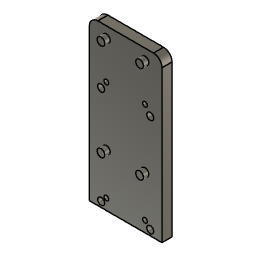
scope-strut-flange v6 (Autodesk Fusion 360 design; units mm, degrees)
Autodesk Fusion 360 part; units mm, degrees
note: some values were not read from the file. Set by a fixed rule: which sketch regions a step uses.
sketch "Sketch1" plane through (0, 0, 0) normal (0, 1, 0) x (1, 0, 0)
  line L0 (47, -103.5) -> (-36, -103.5)
  line L1 (-47, -103.5) -> (-47, 103.5)
  line L2 (-47, 103.5) -> (47, 103.5)
  line L3 (47, 103.5) -> (47, -103.5)
  line L4 (47, -103.5) -> (-47, 103.5) construction
  line L5 (-47, -103.5) -> (47, 103.5) construction
  line L6 (-47, -103.5) -> (36, -103.5)
  line L7 (47, -92.5) -> (47, 96.5)
  line L8 (47, 96.5) -> (-47, 96.5)
  line L9 (-47, 96.5) -> (-47, -92.5)
  line L10 (0, 96.5) -> (-31.75, 96.5)
  line L11 (-31.75, 96.5) -> (31.75, 96.5)
  line L12 (31.75, 96.5) -> (31.75, -30.5)
  line L13 (31.75, -30.5) -> (-31.75, -30.5)
  line L14 (-31.75, -30.5) -> (-31.75, 96.5)
  circle A0 centre (31.75, -30.5) radius 2.05
  circle A1 centre (-31.75, -30.5) radius 2.05
  circle A2 centre (31.75, 96.5) radius 2.05
  circle A3 centre (-31.75, 96.5) radius 2.05
  arc A4 (-47, -92.5) -> (-36, -103.5) centre (-36, -92.5) ccw
  arc A5 (36, -103.5) -> (47, -92.5) centre (36, -92.5) ccw
  point P0 (47, -103.5)
  dimension "d1" = 94
  dimension "d2" = 207
  dimension "d3" = 94
  dimension "d4" = 200
  dimension "d5" = 31.75
  dimension "d6" = 63.5
  dimension "d7" = 127
  dimension "d8" = 4.1
  dimension "d9" = 4.1
  dimension "d10" = 4.1
  dimension "d11" = 4.1
  dimension "d12" = 11
  constraint horizontal L0
  constraint perpendicular L0 L1
  constraint parallel L0 L2
  constraint parallel L1 L3
  constraint coincident L4 origin
  constraint coincident L5 origin
  constraint horizontal L6
  constraint vertical L7
  constraint horizontal L8
  constraint vertical L9
  constraint midpoint L8 L10.start
  constraint perpendicular L1 L10
  constraint horizontal L11
  constraint vertical L12
  constraint horizontal L13
  constraint vertical L14
  constraint coincident L12.end L13.start
  constraint coincident L13.end L14.start
  constraint coincident L11.end L12.start
  constraint coincident L10.end L11.start
  constraint coincident L1.start L0
  constraint coincident L1.start L9
  constraint tangent L0 A4
  constraint tangent L9 A4
  constraint coincident P0 L6
  constraint coincident P0 L7
  constraint tangent L6 A5
  constraint tangent L7 A5
  constraint equal A4 A5
  measures "d1" distance of L1.end L2.end
  measures "d2" distance of L1.start L1.end
  measures "d3" distance of L1.start P0
  measures "d4" distance of L1.start L8.end
  measures "d5" distance of L10.start L10.end
  measures "d6" distance of L10.end L11.end
  measures "d7" distance of L10.end L13.end
  measures "d8" diameter of A0
  measures "d9" diameter of A1
  measures "d10" diameter of A2
  measures "d11" diameter of A3
  measures "d12" radius of A4
extrude "Extrude1" add sketch "Sketch1" along normal blind 10 contours L0 L1 L3 L6 L7 L8 L9 L12 L13 L14 A0 A1 A2 A3 A4 A5 | L1 L2 L3 L8 L10 L11 A2 A3 | L8 L10 L11 L12 L13 L14 A0 A1 A2 A3
sketch "Sketch2" plane through (0, 0, 0) normal (0, -1, 0) x (1, 0, 0)
  circle A0 centre (31.75, -96.5) radius 2.05
  circle A1 centre (-31.75, -96.5) radius 2.05
  circle A2 centre (31.75, 30.5) radius 2.05
  circle A3 centre (-31.75, 30.5) radius 2.05
  line L0 (-47, 92.5) -> (-47, -103.5)
  line L1 (-47, -103.5) -> (47, -103.5)
  line L2 (47, -103.5) -> (47, 92.5)
  arc A4 (47, 92.5) -> (36, 103.5) centre (36, 92.5) ccw
  line L3 (36, 103.5) -> (-36, 103.5)
  arc A5 (-36, 103.5) -> (-47, 92.5) centre (-36, 92.5) ccw
  circle A6 centre (-31.75, 30.5) radius 4.5
  circle A7 centre (31.75, 30.5) radius 4.5
  circle A8 centre (-31.75, -96.5) radius 4.5
  circle A9 centre (31.75, -96.5) radius 4.5
  dimension "d15" = 9
  dimension "d16" = 9
  dimension "d17" = 9
  dimension "d18" = 9
  constraint concentric A3 A6
  constraint concentric A2 A7
  constraint concentric A1 A8
  constraint concentric A0 A9
  measures "d15" diameter of A6
  measures "d16" diameter of A7
  measures "d17" diameter of A8
  measures "d18" diameter of A9
extrude "Extrude2" cut sketch "Sketch2" against normal blind 5 contours A6 | A7 | A8 | A9
sketch "Sketch3" plane through (0, 10, 0) normal (0, 1, 0) x (-1, 0, 0)
  circle A0 centre (-31.75, -96.5) radius 2.05
  circle A1 centre (31.75, -96.5) radius 2.05
  circle A2 centre (-31.75, 30.5) radius 2.05
  circle A3 centre (31.75, 30.5) radius 2.05
  line L0 (47, -103.5) -> (47, 92.5)
  arc A4 (47, 92.5) -> (36, 103.5) centre (36, 92.5) ccw
  line L1 (36, 103.5) -> (-36, 103.5)
  arc A5 (-36, 103.5) -> (-47, 92.5) centre (-36, 92.5) ccw
  line L2 (-47, 92.5) -> (-47, -103.5)
  line L3 (-47, -103.5) -> (47, -103.5)
  line L4 (-47, 103.5) -> (47, 103.5)
  line L5 (47, 103.5) -> (47, 48.5)
  line L6 (47, 48.5) -> (-47, 48.5)
  line L7 (-47, 48.5) -> (-47, 103.5)
  line L8 (-47, 103.5) -> (47, 103.5)
  line L9 (47, 103.5) -> (47, 18.5)
  line L10 (47, 18.5) -> (-47, 18.5)
  line L11 (-47, 18.5) -> (-47, 103.5)
  line L12 (-47, 103.5) -> (47, 103.5)
  line L13 (47, 103.5) -> (47, -89.5)
  line L14 (47, -89.5) -> (-47, -89.5)
  line L15 (-47, -89.5) -> (-47, 103.5)
  line L16 (-47, 48.5) -> (-47, 18.5)
  line L17 (-47, 48.5) -> (47, 18.5)
  line L18 (0, 33.5) -> (0, 40.5)
  line L19 (0, 40.5) -> (25, 40.5)
  line L20 (19.9, 37.5555) -> (25, 34.611)
  line L21 (25, 34.611) -> (30.1, 37.5555)
  line L22 (30.1, 37.5555) -> (30.1, 43.4445)
  line L23 (30.1, 43.4445) -> (25, 46.389)
  line L24 (25, 46.389) -> (19.9, 43.4445)
  line L25 (19.9, 43.4445) -> (19.9, 37.5555)
  line L26 (-25, 46.389) -> (-19.9, 43.4445)
  line L27 (-30.1, 43.4445) -> (-25, 46.389)
  line L28 (-30.1, 37.5555) -> (-30.1, 43.4445)
  line L29 (-25, 34.611) -> (-30.1, 37.5555)
  line L30 (-19.9, 37.5555) -> (-25, 34.611)
  line L31 (-19.9, 43.4445) -> (-19.9, 37.5555)
  circle A6 centre (25, 40.5) radius 3.1
  circle A7 centre (-25, 40.5) radius 3.1
  circle A8 centre (25, -89.5) radius 3.1
  circle A9 centre (-25, -89.5) radius 3.1
  line L32 (19.9, -92.4445) -> (25, -95.389)
  line L33 (25, -95.389) -> (30.1, -92.4445)
  line L34 (30.1, -92.4445) -> (30.1, -86.5555)
  line L35 (30.1, -86.5555) -> (25, -83.611)
  line L36 (25, -83.611) -> (19.9, -86.5555)
  line L37 (19.9, -86.5555) -> (19.9, -92.4445)
  line L38 (-19.9, -86.5555) -> (-25, -83.611)
  line L39 (-25, -83.611) -> (-30.1, -86.5555)
  line L40 (-30.1, -86.5555) -> (-30.1, -92.4445)
  line L41 (-30.1, -92.4445) -> (-25, -95.389)
  line L42 (-25, -95.389) -> (-19.9, -92.4445)
  line L43 (-19.9, -92.4445) -> (-19.9, -86.5555)
  point P0 (25, 40.5)
  point P1 (25, -89.5)
  point P2 (-25, -89.5)
  dimension "d21" = 55
  dimension "d22" = 85
  dimension "d23" = 193
  dimension "d27" = 7
  dimension "d28" = 25
  dimension "d29" = 5.1
  dimension "d30" = 6.2
  dimension "d31" = 6.2
  dimension "d48" = 6.2
  dimension "d49" = 5.1
  dimension "d50" = 5.1
  constraint horizontal L4
  constraint vertical L5
  constraint horizontal L6
  constraint vertical L7
  constraint horizontal L8
  constraint vertical L9
  constraint horizontal L10
  constraint vertical L11
  constraint horizontal L12
  constraint vertical L13
  constraint horizontal L14
  constraint vertical L15
  constraint vertical L18
  constraint midpoint L17 L18.start
  constraint perpendicular L18 L19
  constraint coincident P0 L19.end
  constraint symmetric L18 L20.start L30.start
  constraint symmetric L18 L20.end L29.start
  constraint symmetric L18 L21.end L28.start
  constraint symmetric L18 L22.end L27.start
  constraint symmetric L18 L23.end L26.start
  constraint symmetric L18 L24.end L26.end
  constraint symmetric L18 A6 A7
  constraint coincident P1 A8.centre
  constraint coincident P2 A9.centre
  measures "d21" distance of L4.start L6.end
  measures "d22" distance of L4.start L10.end
  measures "d23" distance of L4.start L14.end
  measures "d27" distance of L18.start L18.end
  measures "d28" distance of L18.end P0
  measures "d29" distance of P0 L25
  measures "d30" diameter of A6
  measures "d31" diameter of A8
  measures "d48" diameter of A9
  measures "d49" distance of P1 L37
  measures "d50" distance of P2 L43
extrude "Extrude3" cut sketch "Sketch3" against normal blind 50.493 contours L14 A8 | L14 A8 | L14 A9 | L14 A9 | L17 A7 | L17 A7 | A6
extrude "Extrude4" cut sketch "Sketch3" against normal blind 5 contours L14 A8 L32 L33 L34 L37 | L14 A8 L34 L35 L36 L37 | L14 A8 | L14 A8 | L14 A9 L38 L39 L40 L43 | L14 A9 L40 L41 L42 L43 | L17 L28 L29 L30 L31 A7 | L17 L26 L27 L28 L31 A7 | L14 A9 | L14 A9 | L20 L21 L22 L23 L24 L25
sketch "Sketch4" plane through (0, 0, 0) normal (0, -1, 0) x (1, 0, 0)
  circle A0 centre (-25, -89.5) radius 3.1
  circle A1 centre (25, 40.5) radius 3.1
  circle A2 centre (25, -89.5) radius 3.1
  circle A3 centre (-25, 40.5) radius 3.1
  circle A4 centre (31.75, -96.5) radius 4.5
  circle A5 centre (-31.75, 30.5) radius 4.5
  circle A6 centre (-31.75, -96.5) radius 4.5
  circle A7 centre (31.75, 30.5) radius 4.5
  line L0 (-47, 92.5) -> (-47, -103.5)
  line L1 (-47, -103.5) -> (47, -103.5)
  line L2 (47, -103.5) -> (47, 92.5)
  arc A8 (47, 92.5) -> (36, 103.5) centre (36, 92.5) ccw
  line L3 (36, 103.5) -> (-36, 103.5)
  arc A9 (-36, 103.5) -> (-47, 92.5) centre (-36, 92.5) ccw
  line L4 (-47, 103.5) -> (47, 103.5)
  line L5 (47, 103.5) -> (47, 89.5)
  line L6 (47, 89.5) -> (-47, 89.5)
  line L7 (-47, 89.5) -> (-47, 103.5)
  line L8 (0, 89.5) -> (-25, 89.5)
  circle A10 centre (-25, 89.5) radius 5
  line L9 (-25, 89.5) -> (25, 89.5)
  line L10 (25, 89.5) -> (25, -35.5)
  line L11 (25, -35.5) -> (-25, -35.5)
  line L12 (-25, -35.5) -> (-25, 89.5)
  circle A11 centre (25, 89.5) radius 5
  circle A12 centre (-25, -35.5) radius 5
  circle A13 centre (25, -35.5) radius 5
  point P0 (-47, 103.5)
  dimension "d36" = 94
  dimension "d37" = 14
  dimension "d38" = 25
  dimension "d39" = 10
  dimension "d40" = 50
  dimension "d41" = 125
  dimension "d42" = 10
  dimension "d43" = 10
  dimension "d44" = 10
  constraint horizontal L4
  constraint vertical L5
  constraint horizontal L6
  constraint vertical L7
  constraint coincident P0 L4.start
  constraint midpoint L6 L8.start
  constraint parallel L6 L8
  constraint coincident L8.end A10.centre
  constraint horizontal L9
  constraint vertical L10
  constraint horizontal L11
  constraint vertical L12
  constraint coincident L9.end L10.start
  constraint coincident L11.end L12.start
  constraint coincident L10.end L11.start
  measures "d36" distance of P0 L4.end
  measures "d37" distance of P0 L6.end
  measures "d38" distance of L8.start L8.end
  measures "d39" diameter of A10
  measures "d40" distance of L8.end L9.end
  measures "d41" distance of L8.end L11.end
  measures "d42" diameter of A11
  measures "d43" diameter of A12
  measures "d44" diameter of A13
  measures "d48" diameter of L4.end
extrude "Extrude5" add sketch "Sketch4" along normal blind 10 contours L6 L9 L10 A11 | L6 L10 A11 | L10 L11 A13 | L10 L11 A13 | L6 L9 A11 | L11 L12 A12 | L11 L12 A12 | L6 L8 A10 L9 L12 | L6 L8 A10 L9 | L6 A10 L12
move_face "OffsetFaces1" offset 3 1 faces at (-7.2942, 0, 7.7625)
equation "d5 = ( 63.5 / 2 ) * 1 mm"
